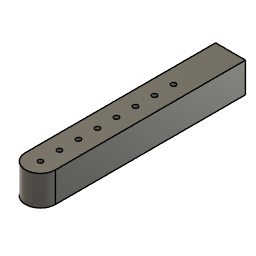
Camera arm 2 v4 (Autodesk Fusion 360 design; units mm, degrees)
Autodesk Fusion 360 part; units mm, degrees
sketch "Sketch1" plane through (0, 0, 0) normal (0, 1, 0) x (1, 0, 0)
  line L0 (20, 0) -> (20, -127)
  line L1 (0, -127) -> (0, 0)
  arc A0 (0, -127) -> (20, -127) centre (10, -127) ccw
  line L2 (0, 0) -> (20, 0)
  circle A1 centre (10, -127) radius 1.6
  dimension "d1" = 20
  dimension "d2" = 127
  dimension "d3" = 3.2
  constraint vertical L0
  constraint vertical L1
  constraint coincident L1.end L2.start
  constraint perpendicular L0 L2
  constraint concentric A0 A1
  measures "d1" distance of L1.end L0.start
  measures "d2" distance of L1.end L1.start
  measures "d3" diameter of A1
extrude "Extrude1" add sketch "Sketch1" along normal blind 20
sketch "Sketch2" plane through (0, 0, 0) normal (0, 0, -1) x (-1, 0, 0)
  line L0 (-20, 0) -> (0, 0)
  line L1 (0, 0) -> (0, 20)
  line L2 (0, 20) -> (-20, 20)
  line L3 (-20, 20) -> (-20, 0)
  line L4 (-20, 20) -> (0, 20)
  line L5 (0, 20) -> (0, 0)
  line L6 (0, 0) -> (-20, 0)
  line L7 (-20, 0) -> (-20, 20)
  circle A0 centre (-16, 16) radius 1
  circle A1 centre (-4, 16) radius 1
  circle A2 centre (-16, 4) radius 1
  circle A3 centre (-4, 4) radius 1
  dimension "d6" = 2
  dimension "d7" = 2
  dimension "d8" = 2
  dimension "d9" = 2
  dimension "d16" = 4
  dimension "d17" = 4
  dimension "d18" = 4
  dimension "d19" = 4
  dimension "d20" = 4
  dimension "d21" = 4
  dimension "d22" = 4
  dimension "d23" = 4
  constraint horizontal L4
  constraint vertical L5
  constraint horizontal L6
  constraint vertical L7
  constraint coincident L0.end L1.start
  constraint coincident L2.end L3.start
  measures "d6" diameter of A0
  measures "d7" diameter of A1
  measures "d8" diameter of A2
  measures "d9" diameter of A3
  measures "d16" distance of L4 A0.centre
  measures "d17" distance of L7 A0.centre
  measures "d18" distance of L4 A1.centre
  measures "d19" distance of L5 A1.centre
  measures "d20" distance of L5 A3.centre
  measures "d21" distance of L6 A3.centre
  measures "d22" distance of L7 A2.centre
  measures "d23" distance of L6 A2.centre
extrude "Extrude2" cut sketch "Sketch2" against normal blind 40 contours A0 | A1 | A2 | A3
sketch "Sketch3" plane through (0, 20, 0) normal (0, 1, 0) x (-1, 0, 0)
  circle A0 centre (-10, 127) radius 1.6
  arc A1 (0, 127) -> (-20, 127) centre (-10, 127) ccw
  line L0 (-20, 127) -> (-20, 0)
  line L1 (-20, 0) -> (0, 0)
  line L2 (0, 0) -> (0, 127)
  circle A2 centre (-10, 114.3) radius 1.6
  circle A3 centre (-10, 101.6) radius 1.6
  circle A4 centre (-10, 88.9) radius 1.6
  circle A5 centre (-10, 76.2) radius 1.6
  circle A6 centre (-10, 63.5) radius 1.6
  circle A7 centre (-10, 50.8) radius 1.6
  circle A8 centre (-10, 38.1) radius 1.6
  dimension "d24" = 3.2
  dimension "d25" = 12.7
  dimension "d28" = 0
  dimension "d29" = -12.7
  measures "d24" diameter of A2
  measures "d25" distance of A0.centre A2.centre
extrude "Extrude3" cut sketch "Sketch3" against normal blind 170 contours A2 | A3 | A4 | A5 | A6 | A7 | A8
